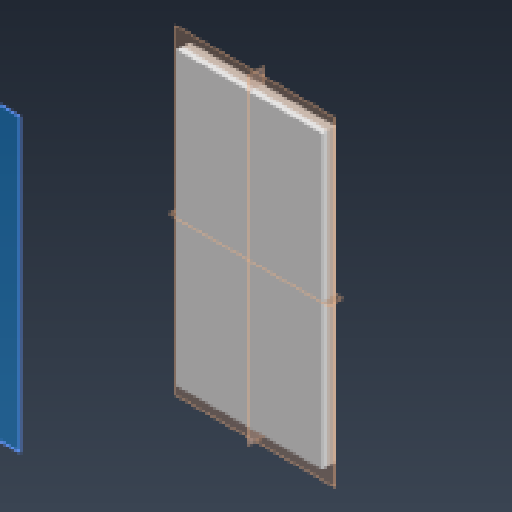
# Autodesk Inventor part: Задняя_крышка
Saved by Autodesk Inventor 2023.2 (Build 272271030, 271C)
## iProperties
Created: 2025-12-13
Part Number: Задняя_крышка
Material: Типовые
Document SubType Name: Modeling
Designer: Олег Коноваленко
Density: 1 g/cm^3
Appearance: По умолчанию
Author: Олег Коноваленко
Autodesk Inventor part; units mm, degrees
sketch "Эскиз1" plane through (0, 0, 0) normal (0, 0, 1) x (1, 0, 0)
  line L0 (-37.5, -100) -> (37.5, -100)
  line L1 (37.5, -100) -> (37.5, 100)
  line L2 (37.5, 100) -> (-37.5, 100)
  line L3 (-37.5, 100) -> (-37.5, -100)
  line L4 (-37.5, -100) -> (37.5, 100) construction
  line L5 (37.5, -100) -> (-37.5, 100) construction
  point P0 (0, 0)
  dimension "d0" = 75
  dimension "d1" = 200
  constraints: 12 end point, 2 midpoint, 2 parallel, 1 horizontal, 1 perpendicular
  measures "d0" distance of L1.end L2.end
  measures "d1" distance of L2.end L0.start
extrude "Выдавливание1" add sketch "Эскиз1" along normal blind 4 and the other way blind 5
